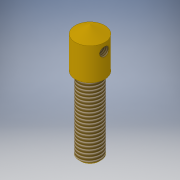
# Autodesk Inventor part: B
Saved by Autodesk Inventor 2017 (Build 210142000, 142)
## iProperties
Part Number: B
Material: 一般
Document SubType Name: Modeling
Designer: user
Density: 1 g/cm^3
Appearance: 金色
Author: user
Autodesk Inventor part; units mm, degrees
ref_plane "YZ Plane" through (0, 0, 0) normal (1, 0, 0) x (0, 1, 0)
ref_plane "XZ Plane" through (0, 0, 0) normal (0, 1, 0) x (-1, 0, 0)
ref_plane "XY Plane" through (0, 0, 0) normal (0, 0, 1) x (1, 0, 0)
sketch "草圖1" plane through (0, 0, 0) normal (0, 0, 1) x (1, 0, 0)
  line L0 (0, 0) -> (6, 0)
  line L1 (6, 0) -> (6, 40)
  line L2 (6, 40) -> (8, 40)
  line L3 (8, 40) -> (8, 57.3812)
  line L4 (0, 62) -> (0, 64.8191)
  line L5 (0, 62) -> (8, 57.3812)
  line L6 (0, 0) -> (0, 62)
  dimension "d0" = 6
  dimension "d1" = 40
  dimension "d3" = 2
  dimension "d6" = 60
  dimension "d7" = 0
  dimension "d8" = 62
  constraints: 14 end point, 2 horizontal, 2 vertical, 1 perpendicular
  measures "d0" distance of L0.start L0.end
  measures "d1" distance of L0.end L1.end
  measures "d3" distance of L1.end L2.end
  measures "d6" angle of L5 L4
  measures "d7" distance from line of L0.start L4
  measures "d8" distance from line of L4.start L0
revolve "迴轉1" add sketch "草圖1" angle 360 about axis through (0, 62, 0) along (0, 1, 0)
chamfer "倒角1" distance 1 distance2 1 1 edges at (-6, 0, 0) measured on face at (-3.0269, 0, 1.5886)
sketch "草圖2" plane through (0, 0, 0) normal (0, -1, 0) x (1, 0, 0)
  circle A0 centre (0, 0) radius 5
  constraints: 1 centre point, 1 coincident
extrude "擠出1" cut sketch "草圖2" against normal blind 36
sketch "草圖4" plane through (0, 0, 0) normal (1, 0, 0) x (0, 1, 0)
  circle A0 centre (53, 0) radius 2.5
  line L0 (40, 8) -> (40, -8) projected
  point P0 (0, 0)
  dimension "d17" = 13
  dimension "d18" = 5
  dimension "d19" = 0
  constraints: 1 centre point
  measures "d17" distance from line of A0.centre L0
  measures "d18" diameter of A0
  measures "d19" vertical distance of point (0, 0) A0.centre
extrude "擠出2" cut sketch "草圖4" along normal through all both and the other way through all
thread "螺紋2" size "M12x1.75" class "6g" standard "ANSI Metric M Profile" full length
thread "螺紋3" size "M6x1" class "6H" standard "ANSI Metric M Profile" full length
